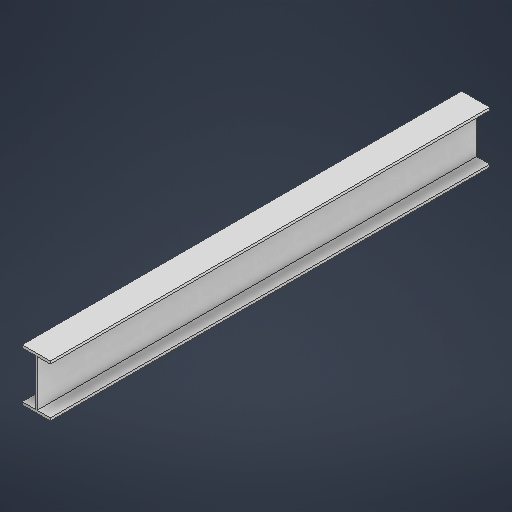
# Autodesk Inventor part: Rail_beam
Saved by Autodesk Inventor 2027.1 (Build 311270010, 270A)
## iProperties
Created: 2026-09-03
Part Number: Rail_beam
Material: Generic
Document SubType Name: Modeling
Designer: ajrcr
Density: 1 g/cm^3
Appearance: Default
Author: ajrcr
Autodesk Inventor part; units mm, degrees
ref_plane "YZ Plane" through (0, 0, 0) normal (1, 0, 0) x (0, 1, 0)
ref_plane "XZ Plane" through (0, 0, 0) normal (0, 1, 0) x (-1, 0, 0)
ref_plane "XY Plane" through (0, 0, 0) normal (0, 0, 1) x (1, 0, 0)
sketch "Sketch1" plane through (0, 0, 0) normal (0, 0, 1) x (1, 0, 0)
  line L0 (0, 0) -> (32, 0)
  line L1 (32, 0) -> (32, 6)
  line L2 (32, 6) -> (2, 6)
  line L3 (2, 6) -> (2, 112)
  line L4 (2, 112) -> (32, 112)
  line L5 (32, 112) -> (32, 118)
  line L6 (32, 118) -> (0, 118)
  line L7 (0, 118) -> (0, 0) construction
  line L8 (0, 0) -> (-32, 0)
  line L9 (-32, 0) -> (-32, 6)
  line L10 (-32, 6) -> (-2, 6)
  line L11 (-2, 6) -> (-2, 112)
  line L12 (-2, 112) -> (-32, 112)
  line L13 (-32, 112) -> (-32, 118)
  line L14 (-32, 118) -> (0, 118)
  dimension "d0" = 6
  dimension "d1" = 2
  dimension "d2" = 6
  dimension "d3" = 32
  dimension "d4" = 118
  dimension "d5" = 32
  constraints: 30 end point, 6 symmetric about line, 5 perpendicular, 1 horizontal, 1 parallel, 1 vertical
  measures "d0" distance of L0.end L1.end
  measures "d1" distance between parallel lines of L7 L3
  measures "d2" distance of L4.end L5.end
  measures "d3" distance of L5.end L6.end
  measures "d4" distance of L6.end L0.start
  measures "d5" distance of L0.start L0.end
extrude "Extrusion1" add sketch "Sketch1" along normal blind 1000
body "Solid1"
